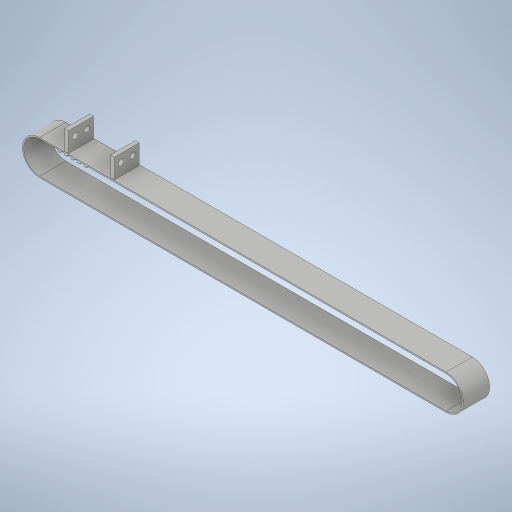
# Autodesk Inventor part: ATBT-700T5200-B-P35_info-1-16-16
Saved by Autodesk Inventor 2023 (Build 270158000, 158)
## iProperties
Category: PARTsolutions
Company: MISUMI
Created: 2023-11-07
Part Number: ATBT-700T5200-B-P35_info-1-16-16
Material: Generic
Catalog Web Link: www.cadenas.de
Description: ATBT-Timing Belts with Attachments-T5, T10 Type
Vendor: MISUMI
Document SubType Name: Modeling
Designer: psAdmin
Manufacturer: MISUMI
Mass: 15.7637 g
Surface Area: 310.297 cm^2
Volume: 15.7637 cm^3
Density: 1 g/cm^3
Appearance: PSOLRGB-175-175-175
PSOL_IDENT_0: {$CADENAS_DATA/23d-libs/misumi/metric/48_timing_belts/atbt.prj},230 {VTYP=3D},{NB=ATBT-700T5200-B-P3
PSOL_IDENT_1: 5_info-1-16-16},{LINA=ATBT-700T5200-B-P35},{NN=ATBT},{DATE=29.05.2023 08:51:55},{GEOMDATE=15.01.2020
PSOL_IDENT_2: 10:09:41},{VERSION=},{LINEID=10},{WBVAR=BCL,BW,ATS,P,RSSP,NT1,NT2},{WBNUMERIC=BCL,BW,P,NT1,NT2}  {N
PSOL_IDENT_3: B=ATBT-700T5200-B-P35_info-1-16-16},{LINA=ATBT-700T5200-B-P35},{KT=DUMMY},{PN=ATBT-700T5200-B-P35},{
PSOL_IDENT_4: TYPE=ATBT},{PS=T5},{BCL=700},{BCLALG=[700:4000/35]},{TNW=200},{BW=20},{BNW1=10,15,20,25},{ATS=B},{AT
PSOL_IDENT_5: SALG='A', 'A', 'B', 'B'},{P=35},{PALG=[30:4000/5]},{P1=20.000},{P2=20},{PMAX=700},{PITCH=5},{NT=140}
PSOL_IDENT_6: ,{RSSP=1},{NT1=16},{NT2=16},{H=2.2},{HH=1.2},{L=1.8},{A=19},{B=15.0},{T=3.0},{DD=4.5},{G=9.0},{F=5},
PSOL_IDENT_7: {C=0.0},{D=0.0},{E=0.0},{K=0.0},{N=0.0},{BNO=700T5},{X=0},{DRIVEP=25.46479},{DRIVENP=25.46479},{DRP=
PSOL_IDENT_8: 24.6},{DRNP=24.6},{PDMAX=25},{PDMIN=25},{RSSP1= '1', '900 or Less', '2', 'Over 900, 1200 or Less', '
PSOL_IDENT_9: 3'  , 'Over 1200, 1800 or Less', '4', 'Over 1800, 3600 or Less', '5'  , 'Over 3600, 4800 or Less' },
PSOL_IDENT_10: {C1=310.00},{BB=1240},{NT1A=12,14,15,16,18,20,22,24,25,26,28,30},{NT2A=16,18,20,22,24,25,26,28,30,32
PSOL_IDENT_11: ,34,36,40,44,48,50,60},{ANG=0.000000},{X2=0},{X3=20},{LUK=40},{LUK1=-255},{ANGROT=-1141.439358},{Z=1
PSOL_IDENT_12: },{Z1=310},{L11=0},{L21=0},{ANG1=247.400421},{FS=32},{FL=32},{DEG1=0},{L3D1=0.75},{L3D2=0.36},{PPN=-
PSOL_IDENT_13: P35},{PPLT=0}
NB: ATBT-700T5200-B-P35_info-1-16-16
NN: ATBT
NT: 140
NBSYN: $PN._info-$RSSP.-$NT1.-$NT2.
LINA: ATBT-700T5200-B-P35
CATALOG: Misumi
PN: ATBT-700T5200-B-P35
TYPE: ATBT
PS: T5
BCL: 700
TNW: 200
BW: 20
ATS: B
P: 35
PITCH: 5
RSSP: 900 or Less
NT1: 16
NT2: 16
H: 2.2
HH: 1.2
L: 1.8
A: 19
B: 15
T: 3
DD: 4.5
G: 9
F: 5
C: 0
D: 0
E: 0
K: 0
N: 0
SUPPLIER: MISUMI
ARTICLENO: ATBT-700T5200-B-P35_info-1-16-16
BOMINFO: ATBT-700T5200-B-P35
CREATOR: CADENAS GmbH
Title: ATBT-700T5200-B-P35
Author: Cadenas PARTsolutions
Comments: Timing Belts with Attachments-T5, T10 Type
Autodesk Inventor part; units mm, degrees
ref_plane "XZ Plane" through (0, 0, 0) normal (0, 1, 0) x (-1, 0, 0)
ref_plane "XY Plane" through (0, 0, 0) normal (0, 0, 1) x (1, 0, 0)
sketch "Sketch_2" plane through (0, 0, 0) normal (0, 0, 1) x (1, 0, 0)
  arc A0 (-20, 13.3) -> (-20, -13.3) centre (-20, 0) ccw
  line L0 (-20, -13.3) -> (290, -13.3)
  arc A1 (290, -13.3) -> (290, 13.3) centre (290, 0) ccw
  line L1 (290, 13.3) -> (-20, 13.3)
  constraints: 4 end point, 4 point on circle, 2 centre point
extrude "Extrusion1" add sketch "Sketch_2" along normal mid plane 20
sketch "Sketch_8" plane through (0, 0, 0) normal (0, 0, 1) x (1, 0, 0)
  line L0 (-1.5, 28.3) -> (-1.5, 13.3)
  line L1 (-1.5, 13.3) -> (1.5, 13.3)
  line L2 (1.5, 13.3) -> (1.5, 28.3)
  line L3 (1.5, 28.3) -> (-1.5, 28.3)
  constraints: 8 end point
extrude "Extrusion2" add sketch "Sketch_8" along normal mid plane 19
sketch "_____4" plane through (0, 0, 0) normal (1, 0, 0) x (0, 0, -1)
  circle A0 centre (-4.5, 22.3) radius 2.25
  constraints: 1 centre point
extrude "Extrusion3" cut sketch "_____4" along normal mid plane 6
sketch "_____5" plane through (0, 0, 0) normal (1, 0, 0) x (0, 0, -1)
  circle A0 centre (4.5, 22.3) radius 2.25
  constraints: 1 centre point
extrude "Extrusion4" cut sketch "_____5" along normal mid plane 6
sketch "_____2" plane through (0, 0, 0) normal (0, 0, 1) x (1, 0, 0)
  line L0 (33.5, 8.3) -> (36.5, 8.3)
  line L1 (36.5, 8.3) -> (36.5, 28.3)
  line L2 (36.5, 28.3) -> (33.5, 28.3)
  line L3 (33.5, 28.3) -> (33.5, 8.3)
  constraints: 8 end point
extrude "Extrusion5" add sketch "_____2" along normal mid plane 19
sketch "Sketch6" plane through (33.5, 13.3, 9.5) normal (-1, 0, 0) x (0, 0, 1)
  point P0 (-14, 9)
hole "Hole1" at (33.5, 22.3, -4.5) direction (1, 0, 0) diameter 4.5 depth 3
sketch "Sketch7" plane through (33.5, 13.3, 9.5) normal (-1, 0, 0) x (0, 0, 1)
  point P0 (-5, 9)
hole "Hole2" at (33.5, 22.3, 4.5) direction (1, 0, 0) diameter 4.5 depth 3
sketch "Sketch_4" plane through (0, 0, 0) normal (0, 0, 1) x (1, 0, 0)
  arc A0 (-20, 12.3) -> (-20, -12.3) centre (-20, 0) ccw
  line L0 (-20, -12.3) -> (290, -12.3)
  arc A1 (290, -12.3) -> (290, 12.3) centre (290, 0) ccw
  line L1 (290, 12.3) -> (17.5, 12.3)
  line L2 (17.5, 12.3) -> (17.5, 11.1)
  line L3 (17.5, 11.1) -> (-7.5, 11.1)
  line L4 (-7.5, 11.1) -> (-7.5, 12.3)
  line L5 (-7.5, 12.3) -> (-20, 12.3)
  constraints: 12 end point, 4 point on circle, 2 centre point
extrude "Extrusion6" cut sketch "Sketch_4" along normal mid plane 20
sketch "Sketch_64" plane through (0, 0, 0) normal (0, 0, 1) x (1, 0, 0)
  line L0 (-9.3801, 11.1) -> (-9.3801, 10.1)
  line L1 (-9.3801, 10.1) -> (-5.6199, 10.1)
  line L2 (-5.6199, 10.1) -> (-5.6199, 11.1)
  arc A0 (-5.9958, 11.3632) -> (-5.6199, 11.1) centre (-5.6199, 11.5) ccw
  line L3 (-5.9958, 11.3632) -> (-6.241, 12.0368)
  arc A1 (-6.241, 12.0368) -> (-6.6168, 12.3) centre (-6.6168, 11.9) ccw
  line L4 (-6.6168, 12.3) -> (-7.125, 12.3)
  line L5 (-7.125, 12.3) -> (-7.125, 12.66)
  line L6 (-7.125, 12.66) -> (-7.875, 12.66)
  line L7 (-7.875, 12.66) -> (-7.875, 12.3)
  line L8 (-7.875, 12.3) -> (-8.3832, 12.3)
  arc A2 (-8.3832, 12.3) -> (-8.759, 12.0368) centre (-8.3832, 11.9) ccw
  line L9 (-8.759, 12.0368) -> (-9.0042, 11.3632)
  arc A3 (-9.3801, 11.1) -> (-9.0042, 11.3632) centre (-9.3801, 11.5) ccw
  constraints: 20 end point, 8 point on circle, 4 centre point
extrude "Extrusion7" cut sketch "Sketch_64" along normal mid plane 20
pattern_linear "Rectangular Pattern1" count 6 spacing 5 along (1, 0, 0) of "Extrusion7"
ref_plane "作業平面3" through (135, 0, 0) normal (1, 0, 0) x (0, 1, 0)
ref_plane "作業平面1" through (303.3, 0, 0) normal (1, 0, 0) x (0, 1, 0)
ref_plane "作業平面2" through (-33.3, 0, 0) normal (1, 0, 0) x (0, 1, 0)
body "Solid1"
